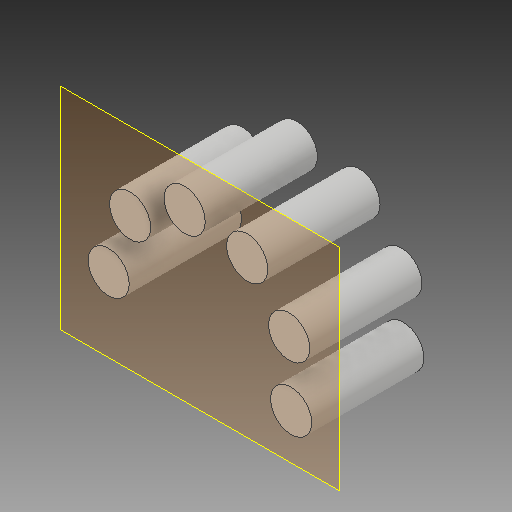
# Autodesk Inventor part: create hole in pelvis
Saved by Autodesk Inventor 2019.3 (Build 233278000, 278)
## iProperties
Created: 2018-10-09
Part Number: create hole in pelvis
Material: Generic
Document SubType Name: Modeling
Designer: HIVE
Density: 1 g/cm^3
Appearance: Default
Author: HIVE
Autodesk Inventor part; units mm, degrees
ref_plane "YZ Plane" through (0, 0, 0) normal (1, 0, 0) x (0, 1, 0)
ref_plane "XZ Plane" through (0, 0, 0) normal (0, 1, 0) x (-1, 0, 0)
ref_plane "XY Plane" through (0, 0, 0) normal (0, 0, 1) x (1, 0, 0)
ref_plane "Work Plane1" through (0, 0, 0) normal (0, 0, 1) x (1, 0, 0)
sketch "Sketch1" plane through (0, 0, 0) normal (0, 0, 1) x (1, 0, 0)
  circle A0 centre (48.7764, -7.7254) radius 5.5 projected
  circle A1 centre (48.2444, 9.2031) radius 5.5 projected
  circle A2 centre (37.0438, 21.9077) radius 5.5 projected
  circle A3 centre (20.3155, 24.5572) radius 5.5 projected
  circle A4 centre (5.7372, 15.9356) radius 5.5 projected
  circle A5 centre (0, 0) radius 5.5 projected
  arc A6 (-1.1822, 9.4262) -> (6.9193, 6.5094) centre (0, 0) ccw projected
  arc A7 (6.9193, 6.5094) -> (15.2179, 16.5407) centre (5.7372, 15.9356) ccw projected
  arc A8 (15.2179, 16.5407) -> (28.0062, 18.9802) centre (20.3155, 24.5572) ccw projected
  arc A9 (28.0062, 18.9802) -> (39.4147, 12.7083) centre (37.0438, 21.9077) ccw projected
  arc A10 (39.4147, 12.7083) -> (44.2073, 0.6036) centre (48.2444, 9.2031) ccw projected
  arc A11 (44.2073, 0.6036) -> (52.8136, 0.8741) centre (48.7764, -7.7254) ccw projected
  arc A12 (52.8136, 0.8741) -> (45.8736, 18.4025) centre (48.2444, 9.2031) ccw projected
  arc A13 (45.8736, 18.4025) -> (29.3531, 27.4847) centre (37.0438, 21.9077) ccw projected
  arc A14 (29.3531, 27.4847) -> (10.8348, 23.9521) centre (20.3155, 24.5572) ccw projected
  arc A15 (10.8348, 23.9521) -> (-1.1822, 9.4262) centre (5.7372, 15.9356) ccw projected
  point P0 (0, 0)
extrude "Extrusion1" add sketch "Sketch1" against normal blind 30 contours A0 | A1 | A2 | A3 | A4 | A5
body "Solid1"
